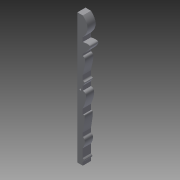
# Autodesk Inventor part: Nozzle
Saved by Autodesk Inventor 2015 (Build 190159000, 159)
## iProperties
Created: 2019-01-10
Part Number: Nozzle
Material: Типовые
Document SubType Name: Modeling
Designer: kostya
Density: 1 g/cm^3
Appearance: По умолчанию
Author: kostya
Autodesk Inventor part; units mm, degrees
ref_plane "YZ Plane" through (0, 0, 0) normal (1, 0, 0) x (0, 1, 0)
ref_plane "XZ Plane" through (0, 0, 0) normal (0, 1, 0) x (-1, 0, 0)
ref_plane "XY Plane" through (0, 0, 0) normal (0, 0, 1) x (1, 0, 0)
sketch "Эскиз1" plane through (0, 0, 0) normal (0, 0, 1) x (1, 0, 0)
  line L0 (-5, -7.5) -> (5, -7.5)
  line L1 (5, -7.5) -> (5, 7.5)
  line L2 (5, 7.5) -> (-5, 7.5)
  line L3 (-5, 7.5) -> (-5, -7.5)
  line L4 (-5, -7.5) -> (5, 7.5) construction
  line L5 (5, -7.5) -> (-5, 7.5) construction
  point P0 (0, 0)
  dimension "d0" = 10
  dimension "d1" = 15
  constraints: 12 end point, 2 midpoint, 2 parallel, 1 horizontal, 1 perpendicular
  measures "d0" distance of L2.end L1.end
  measures "d1" distance of L1.end L0.end
extrude "Выдавливание1" add sketch "Эскиз1" along normal mid plane 240
sketch "Эскиз3" plane through (-5, 7.5, 120) normal (0, 1, 0) x (1, 0, 0)
  line L0 (10, 0) -> (22.4133, 11.0717) construction
  line L1 (10, 240) -> (10, 0) projected
  line L2 (18.7544, 123.2595) -> (14.9087, 136.6513) construction
  line L3 (14.9087, 136.6513) -> (10, 148.7613) construction
  line L4 (12.2217, 156.9873) -> (15.1095, 158.4366) construction
  line L5 (10, 158.6272) -> (12.2217, 156.9873) construction
  spline S0 degree 4 poles (10, 120.3104) (10.6885, 120.4) (14.5524, 120.9622) (18.7544, 123.2595) (14.9087, 136.6513) (10, 148.7613) knots 7.806725 7.806725 7.806725 7.806725 7.806725 8 8.816044 8.816044 8.816044 8.816044 8.816044
  line L6 (16.1722, 104.0435) -> (12.6846, 108.5719) construction
  line L7 (12.6846, 108.5719) -> (10, 112.3423) construction
  line L8 (14.5524, 120.9622) -> (18.7544, 123.2595) construction
  line L9 (10.6885, 120.4) -> (14.5524, 120.9622) construction
  line L10 (10, 120.3104) -> (10.6885, 120.4) construction
  line L11 (19.5701, 51.9157) -> (11.8452, 59.5335) construction
  line L12 (11.8452, 59.5335) -> (10, 61.4441) construction
  line L13 (12.6625, 64.9164) -> (17.1948, 66.8214) construction
  line L14 (10, 64.7616) -> (12.6625, 64.9164) construction
  spline S1 degree 4 poles (10, 0) (22.4133, 11.0717) (20.5125, 21.2759) (14.9788, 29.1456) (10, 34.6409) knots 1 1 1 1 1 1.479533 1.479533 1.479533 1.479533 1.479533
  spline S2 degree 4 poles (10, 42.4578) (17.8063, 40.9171) (31.518, 38.9171) (19.5701, 51.9157) (11.8452, 59.5335) (10, 61.4441) knots 2.157548 2.157548 2.157548 2.157548 2.157548 3 3.460409 3.460409 3.460409 3.460409 3.460409
  line L15 (22.4133, 11.0717) -> (20.5125, 21.2759) construction
  line L16 (20.5125, 21.2759) -> (14.9788, 29.1456) construction
  line L17 (14.9788, 29.1456) -> (10, 34.6409) construction
  line L18 (31.518, 38.9171) -> (19.5701, 51.9157) construction
  line L19 (17.8063, 40.9171) -> (31.518, 38.9171) construction
  line L20 (10, 42.4578) -> (17.8063, 40.9171) construction
  spline S3 degree 4 poles (10, 64.7616) (12.6625, 64.9164) (17.1948, 66.8214) (12.7242, 81.5872) (10.4023, 92.5211) (10, 95.1158) knots 4.079114 4.079114 4.079114 4.079114 4.079114 5 5.351232 5.351232 5.351232 5.351232 5.351232
  spline S4 degree 4 poles (10, 102.7457) (10.3255, 103.6616) (12.3365, 106.1869) (16.1722, 104.0435) (12.6846, 108.5719) (10, 112.3423) knots 5.710697 5.710697 5.710697 5.710697 5.710697 6 6.927418 6.927418 6.927418 6.927418 6.927418
  line L21 (17.1948, 66.8214) -> (12.7242, 81.5872) construction
  line L22 (12.7242, 81.5872) -> (10.4023, 92.5211) construction
  line L23 (10.4023, 92.5211) -> (10, 95.1158) construction
  line L24 (12.3365, 106.1869) -> (16.1722, 104.0435) construction
  line L25 (10.3255, 103.6616) -> (12.3365, 106.1869) construction
  line L26 (10, 102.7457) -> (10.3255, 103.6616) construction
  spline S5 degree 4 poles (10, 158.6272) (12.2217, 156.9873) (15.1095, 158.4366) (12.3637, 173.2023) (10.5216, 183.4118) (10, 187.241) knots 10.452108 10.452108 10.452108 10.452108 10.452108 11 11.609642 11.609642 11.609642 11.609642 11.609642
  line L27 (15.1095, 158.4366) -> (12.3637, 173.2023) construction
  line L28 (12.3637, 173.2023) -> (10.5216, 183.4118) construction
  line L29 (10.5216, 183.4118) -> (10, 187.241) construction
  line L30 (10.7467, 195.0702) -> (13.4688, 194.3249) construction
  line L31 (10, 193.6844) -> (10.7467, 195.0702) construction
  spline S6 degree 4 poles (10, 193.6844) (10.7467, 195.0702) (13.4688, 194.3249) (15.4545, 200.7955) (11.7294, 208.8265) (10, 212.1471) knots 12.053463 12.053463 12.053463 12.053463 12.053463 13 13.695165 13.695165 13.695165 13.695165 13.695165
  spline S7 degree 4 poles (10, 227.67) (10.6941, 228.2247) (12.3194, 229.5337) (13.2597, 230.885) (11.5359, 232.7441) (10, 233.9261) knots 14.764065 14.764065 14.764065 14.764065 14.764065 15 15.335911 15.335911 15.335911 15.335911 15.335911
  line L32 (13.4688, 194.3249) -> (15.4545, 200.7955) construction
  line L33 (15.4545, 200.7955) -> (11.7294, 208.8265) construction
  line L34 (11.7294, 208.8265) -> (10, 212.1471) construction
  line L35 (10.6941, 228.2247) -> (12.3194, 229.5337) construction
  line L36 (10, 227.67) -> (10.6941, 228.2247) construction
  line L37 (12.3194, 229.5337) -> (13.2597, 230.885) construction
  line L38 (13.2597, 230.885) -> (11.5359, 232.7441) construction
  line L39 (11.5359, 232.7441) -> (10, 233.9261) construction
  point P0 (5, 120)
  constraints: 40 other
extrude "Выдавливание3" add sketch "Эскиз3" against normal blind 15
sketch "Эскиз4" plane through (-5, 7.5, -120) normal (0, 1, 0) x (1, 0, 0)
  line L0 (0, -240) -> (0, -120) construction
  line L1 (0, 0) -> (0, -240) construction
  circle A0 centre (5, -120) radius 2
  dimension "d15" = 4
  constraints: 2 end point, 1 centre point, 1 coincident, 1 midpoint
  measures "d15" diameter of A0
extrude "Выдавливание4" cut sketch "Эскиз4" against normal blind 15
